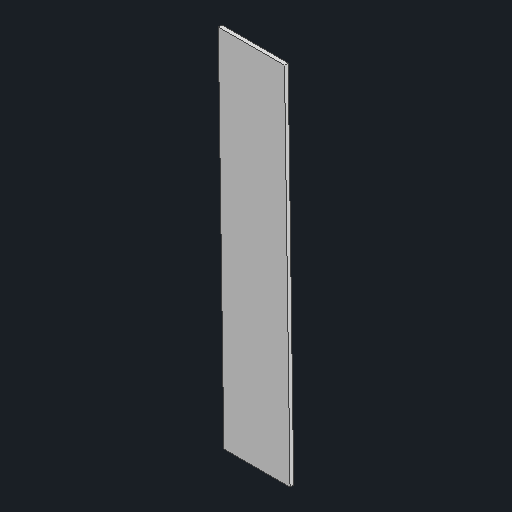
# Autodesk Inventor part: sponson_indent
Saved by Autodesk Inventor 2023 (Build 270158030, 158C)
## iProperties
Created: 2022-03-24
Part Number: sponson_indent
Material: Generic
Document SubType Name: Modeling
Designer: kardo
Density: 1 g/cm^3
Appearance: Default
Author: kardo
Autodesk Inventor part; units mm, degrees
ref_plane "YZ Plane" through (0, 0, 0) normal (1, 0, 0) x (0, 1, 0)
ref_plane "XZ Plane" through (0, 0, 0) normal (0, 1, 0) x (-1, 0, 0)
ref_plane "XY Plane" through (0, 0, 0) normal (0, 0, 1) x (1, 0, 0)
derived "parameters_frame.ipt"
derived "surface_body.ipt"
sketch "sk_long_outer" plane through (0, 0, 0) normal (1, 0, 0) x (0, 1, 0)
  line L0 (-345, 107.6209) -> (-345, -224.5198) construction
  line L1 (255, 107.6209) -> (255, -224.5198) construction
  line L2 (-465, 54.4) -> (375, 54.4) construction
  line L3 (-483, 0) -> (357, 0) construction
  line L4 (0, 107.6209) -> (0, -224.5198) construction
  line L5 (0, 14.144) -> (-345, 11.968)
  line L6 (-345, 11.968) -> (-345, 39.712)
  line L7 (-345, 39.712) -> (0, 54.4)
  line L8 (0, 54.4) -> (255, 36.448)
  line L9 (0, 0) -> (122.4, 9.6331)
  line L10 (122.4, 9.6331) -> (255, 36.448)
  line L11 (0, 14.144) -> (0, 0)
  line L12 (0, 14.144) -> (121.9006, 15.9783)
  line L13 (121.9006, 15.9783) -> (122.4, 9.6331)
sketch "sk_cross" plane through (0, 0, 0) normal (0, 1, 0) x (-1, 0, 0)
  line L0 (0, -224.5198) -> (0, 107.6209) construction
  line L1 (-156, -224.5198) -> (-156, 107.6209) construction
  line L2 (156, -224.5198) -> (156, 107.6209)
  line L3 (-188.7979, 0) -> (31.4663, 0) construction
  line L4 (-188.7979, 54.4) -> (31.4663, 54.4) construction
  line L5 (-81.12, -224.5198) -> (-81.12, 107.6209) construction
  line L6 (-54.6, -224.5198) -> (-54.6, 107.6209) construction
  line L7 (-34.32, -224.5198) -> (-34.32, 107.6209) construction
  line L8 (0, 54.4) -> (-54.6, 54.4)
  line L9 (-54.6, 54.4) -> (-81.12, 52.8758)
  line L10 (-81.12, 0) -> (-81.12, 52.8758)
  line L11 (-81.12, 14.144) -> (-107.2232, 45.2526)
  line L12 (-156, 31.008) -> (-126.048, 0)
  line L13 (-126.048, 0) -> (-81.12, 0)
  line L14 (-81.12, 52.8758) -> (-156, 31.008)
  arc A0 (-54.6, 54.4) -> (-156, 31.008) centre (-54.6, -177.0711) ccw construction
  line L15 (-81.12, 14.144) -> (-102.6854, 14.144)
  line L16 (-102.6854, 14.144) -> (-102.6854, 0)
  point P0 (0, 0)
ref_plane "plane_tunnel_right" through (81.12, 0, 0) normal (1, 0, 0) x (0, 1, 0)
sketch "sk_profile" plane through (81.12, 0, 0) normal (1, 0, 0) x (0, 1, 0)
  line L0 (0, 14.144) -> (119.9008, 15.9482)
  line L1 (119.9008, 15.9482) -> (121.9006, 15.9783) construction
  point P0 (0, 0)
  dimension "d2" = 2
  constraints: 4 end point, 1 collinear
  measures "d2" distance of L0.end L1.end
surface extrude "surface" sketch "sk_profile" along normal up to surface (21.5654 mm away) shown no curves L0
thicken "thicken" operation new thickness 1.2 both sides no extend neighbours no toward (0, -0.0150455, 0.9998868) faces at (88.3085, 39.9669, 14.7454)
equation "\"d2\" = bulkhead_thickness"
equation "\"d5\" = shell_thickness"
equation "\"d6\" = shell_thickness"
equation "\"bulkhead_thickness\" = 2"
equation "\"shell_thickness\" = 1.2"
body "Solid1"
body "Srf1"
